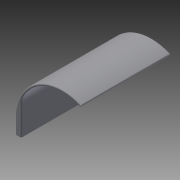
# Autodesk Inventor part: tunel.viento
Saved by Autodesk Inventor 2015 SP1 (Build 190203100, 203)
## iProperties
Created: 2015-07-20
Part Number: tunel.viento
Material: Generic
Document SubType Name: Modeling
Designer: pc
Density: 1 g/cm^3
Appearance: Default
Author: pc
Autodesk Inventor part; units mm, degrees
ref_plane "YZ Plane" through (0, 0, 0) normal (1, 0, 0) x (0, 1, 0)
ref_plane "XZ Plane" through (0, 0, 0) normal (0, 1, 0) x (-1, 0, 0)
ref_plane "XY Plane" through (0, 0, 0) normal (0, 0, 1) x (1, 0, 0)
sketch "Sketch1" plane through (0, 0, 0) normal (0, 0, 1) x (1, 0, 0)
  line L0 (-8, 0) -> (0, 0)
  line L1 (0, 0) -> (0, 120)
  line L2 (0, 120) -> (-8, 120)
  line L3 (-8, 120) -> (-8, 0)
  line L4 (0, 34) -> (-16, 34) construction
  line L5 (-8, 30) -> (-12, 30)
  line L6 (-12, 38) -> (-8, 38)
  arc A0 (-12, 38) -> (-12, 30) centre (-12, 34) ccw
  line L7 (0, 86) -> (-16, 86) construction
  line L8 (-8, 82) -> (-12, 82)
  line L9 (-12, 90) -> (-8, 90)
  arc A1 (-12, 90) -> (-12, 82) centre (-12, 86) ccw
  circle A2 centre (-12, 34) radius 1.75
  circle A3 centre (-12, 86) radius 1.75
  line L10 (0, 60) -> (-8, 60)
  point P0 (-8, 34)
  point P1 (-8, 86)
  dimension "d0" = 8
  dimension "d1" = 120
  dimension "d2" = 52
  dimension "d3" = 3.5
  dimension "d4" = 3.5
  dimension "d5" = 4
  dimension "d6" = 4
  dimension "d7" = 4
  constraints: 25 end point, 6 point on circle, 5 horizontal, 4 centre point, 4 tangent, 3 midpoint, 3 parallel, 2 coincident, 2 point on line, 1 perpendicular, 1 symmetric about line, 1 vertical, 10 other
  measures "d0" distance of L0.end L0.start
  measures "d1" distance of L2.end L0.start
  measures "d2" distance of A1.centre A0.centre
  measures "d3" diameter of A2
  measures "d4" diameter of A3
  measures "d5" radius of A0
  measures "d6" radius of A1
extrude "Extrusion1" add sketch "Sketch1" along normal blind 4
sketch "Sketch2" plane through (-8, 0, 0) normal (0, -1, 0) x (1, 0, 0)
  line L0 (0, 0) -> (8, 0) projected
  line L1 (8, 0) -> (8, 4) projected
  line L2 (0, 4) -> (8, 4) projected
  line L3 (0, 0) -> (0, 4) projected
  line L4 (8, 4) -> (8, 44)
  arc A0 (88.2833, 74.4337) -> (8, 44) centre (63, 20.0208) ccw
  arc A1 (88.2833, 77.7249) -> (0, 20.0208) centre (63, 20.0208) ccw
  line L5 (88.2833, 77.7249) -> (88.2833, 74.4337)
  line L6 (0, 4) -> (0, 20.0208)
  dimension "d10" = 40
  dimension "d11" = 60
  dimension "d20" = 63
  dimension "d22" = 3.2912
  constraints: 6 end point, 4 point on circle, 3 vertical, 2 centre point, 1 coincident, 1 tangent
  measures "d10" distance of L1.end L4.end
  measures "d11" radius of A0
  measures "d20" radius of A1
  measures "d22" distance of L5.start L5.end
extrude "Extrusion2" add sketch "Sketch2" against normal up to surface (120 mm away) from surface at 0 contours L6 A1 L5 A0 L4 L2
fillet "Fillet1" radius 20 1 edges at (0, 60, 44)
fillet "Fillet2" radius 20 4 edges at (-8, 38, 2) (-8, 90, 2) (-8, 82, 2) (-8, 30, 2)
fillet "Fillet3" radius 1.5 12 edges at (-8, 120, 10.0104) (20.5315, 120, 72.7553) (0.6351, 120, 44.3858) (0, 120, 19.6929) (36.3979, 120, 77.0643) (80.2833, 60, 77.7249) (80.2833, 60, 74.4337) (-8, 0, 10.0104) (20.5315, 0, 72.7553) (0.6351, 0, 44.3858) (0, 0, 19.6929) (36.3979, 0, 77.0643)
fillet "Fillet4" radius 2 2 edges at (-8, 34, 4) (-8, 86, 4)
body "Solid1"
